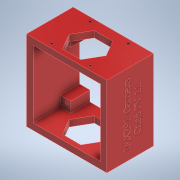
# Autodesk Inventor part: IMX291 Camera Case Base
Saved by Autodesk Inventor 2022.1 (Build 261234000, 234)
## iProperties
Created: 2021-07-23
Part Number: IMX291 Camera Case Base
Material: PET Plastic
Document SubType Name: Modeling
Designer: robst
Density: 1.541 g/cm^3
Appearance: Red
Author: robst
Autodesk Inventor part; units mm, degrees
ref_plane "YZ Plane" through (0, 0, 0) normal (1, 0, 0) x (0, 1, 0)
ref_plane "XZ Plane" through (0, 0, 0) normal (0, 1, 0) x (-1, 0, 0)
ref_plane "XY Plane" through (0, 0, 0) normal (0, 0, 1) x (1, 0, 0)
sketch "Sketch8" plane through (0, 0, 0) normal (0, 0, 1) x (1, 0, 0)
  line L0 (-17, -17) -> (17, -17) construction
  line L1 (17, -17) -> (17, 17) construction
  line L2 (17, 17) -> (-17, 17) construction
  line L3 (-17, 17) -> (-17, -17) construction
  line L4 (-17, -17) -> (17, 17) construction
  line L5 (17, -17) -> (-17, 17) construction
  circle A0 centre (-17, 17) radius 0.9
  circle A1 centre (17, 17) radius 0.9
  circle A2 centre (17, -17) radius 0.9
  circle A3 centre (-17, -17) radius 0.9
  line L6 (-21, -21) -> (21, -21)
  line L7 (21, -21) -> (21, 21)
  line L8 (21, 21) -> (-21, 21)
  line L9 (-21, 21) -> (-21, -21)
  line L10 (-21, -21) -> (21, 21) construction
  line L11 (21, -21) -> (-21, 21) construction
  line L12 (-25, -25) -> (25, -25)
  line L13 (25, -25) -> (25, 25)
  line L14 (25, 25) -> (-25, 25)
  line L15 (-25, 25) -> (-25, -25)
  line L16 (-25, -25) -> (25, 25) construction
  line L17 (25, -25) -> (-25, 25) construction
  line L18 (0, 0) -> (9.8286, 0)
  line L19 (-14.5, -14.5) -> (14.5, -14.5) construction
  line L20 (14.5, -14.5) -> (14.5, 14.5) construction
  line L21 (14.5, 14.5) -> (-14.5, 14.5) construction
  line L22 (-14.5, 14.5) -> (-14.5, -14.5) construction
  line L23 (-14.5, -14.5) -> (14.5, 14.5) construction
  line L24 (14.5, -14.5) -> (-14.5, 14.5) construction
  line L25 (-21, 21) -> (-14.5, 21)
  line L26 (-14.5, 21) -> (-14.5, 14.5)
  line L27 (-14.5, 14.5) -> (-21, 14.5)
  line L28 (-21, 14.5) -> (-21, 21)
  line L29 (21, 21) -> (14.5, 21)
  line L30 (14.5, 21) -> (14.5, 14.5)
  line L31 (14.5, 14.5) -> (21, 14.5)
  line L32 (21, 14.5) -> (21, 21)
  line L33 (21, -21) -> (14.5, -21)
  line L34 (14.5, -21) -> (14.5, -14.5)
  line L35 (14.5, -14.5) -> (21, -14.5)
  line L36 (21, -14.5) -> (21, -21)
  line L37 (-21, -21) -> (-14.5, -21)
  line L38 (-14.5, -21) -> (-14.5, -14.5)
  line L39 (-14.5, -14.5) -> (-21, -14.5)
  line L40 (-21, -14.5) -> (-21, -21)
  point P0 (-25, 0)
  point P1 (-14.5, -21)
  dimension "d46" = 34
  dimension "d47" = 34
  dimension "d48" = 1.8
  dimension "d49" = 42
  dimension "d50" = 42
  dimension "d51" = 4
  dimension "d52" = 4
  dimension "d53" = 29
  dimension "d54" = 29
  dimension "d61" = 50
  dimension "d62" = 50
  constraints: 82 end point, 16 parallel, 9 midpoint, 8 horizontal, 8 perpendicular, 4 centre point, 4 coincident, 3 equal radius, 2 point on line
  measures "d46" distance of L0.start L0.end
  measures "d47" distance of L2.end L0.start
  measures "d48" diameter of A0
  measures "d49" distance of L7.end L8.end
  measures "d50" distance of L6.end L7.end
  measures "d51" distance between parallel lines of L8 L14
  measures "d52" distance from line of point (-25, 0) L9
  measures "d53" distance of L19.start L19.end
  measures "d54" distance of L20.end L19.end
  measures "d61" distance between parallel lines of L14 L12
  measures "d62" distance between parallel lines of L15 L13
extrude "Extrusion9" add sketch "Sketch8" against normal blind 12 contours L9 L39 L38 L6 | L34 L35 L7 L6 | L9 L8 L26 L27 | L31 L30 L8 L7 | L15 L14 L13 L12
sketch "Sketch9" plane through (0, 0, 0) normal (0, 0, 1) x (1, 0, 0)
  line L0 (21, 14.5) -> (21, -14.5) projected
  line L1 (-14.5, 21) -> (14.5, 21) projected
  line L2 (-21, -14.5) -> (-21, 14.5) projected
  line L3 (14.5, -21) -> (-14.5, -21) projected
  line L4 (-25, -25) -> (25, -25) projected
  line L5 (25, -25) -> (25, 25) projected
  line L6 (25, 25) -> (-25, 25) projected
  line L7 (-25, 25) -> (-25, -25) projected
  line L8 (-21, -21) -> (21, -21)
  line L9 (21, -21) -> (21, 21)
  line L10 (21, 21) -> (-21, 21)
  line L11 (-21, 21) -> (-21, -21)
  line L12 (-21, -21) -> (21, 21) construction
  line L13 (21, -21) -> (-21, 21) construction
  line L14 (-23, -23) -> (23, -23)
  line L15 (23, -23) -> (23, 23)
  line L16 (23, 23) -> (-23, 23)
  line L17 (-23, 23) -> (-23, -23)
  line L18 (-23, -23) -> (23, 23) construction
  line L19 (23, -23) -> (-23, 23) construction
  point P0 (0, 0)
  point P1 (-14.5, -21)
  constraints: 24 end point, 4 midpoint, 4 parallel, 2 perpendicular
extrude "Extrusion10" add sketch "Sketch9" along normal blind 17 contours L7 L6 L5 L4 | L17 L16 L15 L14
sketch "Sketch10" plane through (25, -25, -12) normal (1, 0, 0) x (0, 0, -1)
  line L0 (-29, 0) -> (0, 0) construction
  line L1 (-14.5, 0) -> (-14.5, 50) construction
  line L2 (0, 50) -> (-29, 50) construction
  line L3 (-14.5, 7.4068) -> (-14.5, 5.8574)
  line L4 (-14.5, 5.8574) -> (-14.9084, 5.8574)
  line L5 (-14.9084, 5.8574) -> (-14.9084, 6.3663)
  line L6 (-14.9084, 6.3663) -> (-18.0916, 6.3663)
  line L7 (-18.0916, 6.3663) -> (-18.0916, 5.8574)
  line L8 (-18.0916, 5.8574) -> (-18.5, 5.8574)
  line L9 (-18.5, 5.8574) -> (-18.5, 7.4068)
  line L10 (-18.5, 7.4068) -> (-18.0916, 7.4068)
  line L11 (-18.0916, 7.4068) -> (-18.0916, 6.8979)
  line L12 (-18.0916, 6.8979) -> (-14.9084, 6.8979)
  line L13 (-14.9084, 6.8979) -> (-14.9084, 7.4068)
  line L14 (-14.9084, 7.4068) -> (-14.5, 7.4068)
  line L15 (-14.5, 11.4943) -> (-14.5, 10.9627)
  line L16 (-14.5, 10.9627) -> (-17.9457, 10.9627)
  line L17 (-17.9457, 10.9627) -> (-15.6021, 9.919)
  line L18 (-15.6021, 9.919) -> (-15.6021, 9.5948)
  line L19 (-15.6021, 9.5948) -> (-17.9457, 8.5608)
  line L20 (-17.9457, 8.5608) -> (-14.5, 8.5608)
  line L21 (-14.5, 8.5608) -> (-14.5, 8.0648)
  line L22 (-14.5, 8.0648) -> (-18.5, 8.0648)
  line L23 (-18.5, 8.0648) -> (-18.5, 8.7909)
  line L24 (-18.5, 8.7909) -> (-16.2731, 9.7893)
  line L25 (-16.2731, 9.7893) -> (-18.5, 10.7553)
  line L26 (-18.5, 10.7553) -> (-18.5, 11.4943)
  line L27 (-18.5, 11.4943) -> (-14.5, 11.4943)
  line L28 (-14.5, 15.0697) -> (-14.5, 14.4603)
  line L29 (-14.5, 14.4603) -> (-16.0948, 13.4878)
  line L30 (-16.0948, 13.4878) -> (-14.5, 12.4959)
  line L31 (-14.5, 12.4959) -> (-14.5, 11.9222)
  line L32 (-14.5, 11.9222) -> (-16.5032, 13.1961)
  line L33 (-16.5032, 13.1961) -> (-18.5, 11.9611)
  line L34 (-18.5, 11.9611) -> (-18.5, 12.5705)
  line L35 (-18.5, 12.5705) -> (-16.9344, 13.5235)
  line L36 (-16.9344, 13.5235) -> (-18.5, 14.4959)
  line L37 (-18.5, 14.4959) -> (-18.5, 15.0697)
  line L38 (-18.5, 15.0697) -> (-16.5292, 13.8185)
  line L39 (-16.5292, 13.8185) -> (-14.5, 15.0697)
  line L40 (-14.5, 17.8509) -> (-14.5, 15.3841)
  line L41 (-14.5, 15.3841) -> (-15.0673, 15.3841)
  spline S0 degree 2 poles (-15.0673, 15.3841) (-15.3169, 15.6499) (-15.7804, 16.1232) (-16.03, 16.3501) knots 0 0 0 1 2 2 2
  spline S1 degree 2 poles (-16.03, 16.3501) (-16.5324, 16.8071) (-17.1353, 17.141) (-17.4562, 17.141) knots 0 0 0 1 2 2 2
  spline S2 degree 2 poles (-17.4562, 17.141) (-17.6248, 17.141) (-17.8776, 17.0373) (-17.9587, 16.9433) knots 0 0 0 1 2 2 2
  spline S3 degree 2 poles (-17.9587, 16.9433) (-18.0397, 16.8493) (-18.1207, 16.6029) (-18.1207, 16.4538) knots 0 0 0 1 2 2 2
  spline S4 degree 2 poles (-18.1207, 16.4538) (-18.1207, 16.3112) (-18.0494, 16.0194) (-17.9943, 15.8865) knots 0 0 0 1 2 2 2
  spline S5 degree 2 poles (-17.9943, 15.8865) (-17.9489, 15.7731) (-17.8193, 15.5624) (-17.7739, 15.4976) knots 0 0 0 1 2 2 2
  line L42 (-17.7739, 15.4976) -> (-17.7739, 15.4684)
  line L43 (-17.7739, 15.4684) -> (-18.3444, 15.4684)
  spline S6 degree 2 poles (-18.3444, 15.4684) (-18.4254, 15.6337) (-18.5843, 16.2269) (-18.5843, 16.4927) knots 0 0 0 1 2 2 2
  spline S7 degree 2 poles (-18.5843, 16.4927) (-18.5843, 17.0535) (-17.9911, 17.6856) (-17.4854, 17.6856) knots 0 0 0 1 2 2 2
  spline S8 degree 2 poles (-17.4854, 17.6856) (-17.2488, 17.6856) (-16.8533, 17.5754) (-16.6848, 17.4781) knots 0 0 0 1 2 2 2
  spline S9 degree 2 poles (-16.6848, 17.4781) (-16.5097, 17.3809) (-16.1661, 17.0989) (-16.0008, 16.9433) knots 0 0 0 1 2 2 2
  spline S10 degree 2 poles (-16.0008, 16.9433) (-15.7253, 16.6904) (-15.1353, 16.0713) (-14.9635, 15.8865) knots 0 0 0 1 2 2 2
  line L44 (-14.9635, 15.8865) -> (-14.9635, 17.8509)
  line L45 (-14.9635, 17.8509) -> (-14.5, 17.8509)
  spline S11 degree 2 poles (-17.2002, 18.2755) (-17.5081, 18.2755) (-18.0203, 18.4765) (-18.205, 18.6515) knots 0 0 0 1 2 2 2
  spline S12 degree 2 poles (-18.205, 18.6515) (-18.3833, 18.8169) (-18.581, 19.2998) (-18.581, 19.5462) knots 0 0 0 1 2 2 2
  spline S13 degree 2 poles (-18.581, 19.5462) (-18.581, 19.8217) (-18.3963, 20.269) (-18.2212, 20.4344) knots 0 0 0 1 2 2 2
  spline S14 degree 2 poles (-18.2212, 20.4344) (-18.0008, 20.6418) (-17.2877, 20.8687) (-16.7399, 20.8687) knots 0 0 0 1 2 2 2
  spline S15 degree 2 poles (-16.7399, 20.8687) (-16.2439, 20.8687) (-15.3558, 20.6451) (-15.0608, 20.4279) knots 0 0 0 1 2 2 2
  spline S16 degree 2 poles (-15.0608, 20.4279) (-14.7496, 20.1977) (-14.4222, 19.5494) (-14.4222, 19.0762) knots 0 0 0 1 2 2 2
  spline S17 degree 2 poles (-14.4222, 19.0762) (-14.4222, 18.9692) (-14.4449, 18.7261) (-14.4773, 18.6224) knots 0 0 0 1 2 2 2
  line L46 (-14.4773, 18.6224) -> (-14.9927, 18.6224)
  line L47 (-14.9927, 18.6224) -> (-14.9927, 18.6483)
  spline S18 degree 2 poles (-14.9927, 18.6483) (-14.9538, 18.7164) (-14.8857, 19.0016) (-14.8857, 19.1475) knots 0 0 0 1 2 2 2
  spline S19 degree 2 poles (-14.8857, 19.1475) (-14.8857, 19.6726) (-15.5794, 20.2723) (-16.2212, 20.3144) knots 0 0 0 1 2 2 2
  spline S20 degree 2 poles (-16.2212, 20.3144) (-16.0754, 20.1005) (-15.9425, 19.7115) (-15.9425, 19.4814) knots 0 0 0 1 2 2 2
  spline S21 degree 2 poles (-15.9425, 19.4814) (-15.9425, 19.2609) (-16.0397, 18.8947) (-16.1791, 18.7099) knots 0 0 0 1 2 2 2
  spline S22 degree 2 poles (-16.1791, 18.7099) (-16.3444, 18.4959) (-16.8468, 18.2755) (-17.2002, 18.2755) knots 0 0 0 1 2 2 2
  spline S23 degree 2 poles (-16.8598, 20.3274) (-17.265, 20.3274) (-17.7771, 20.1783) (-17.9165, 20.0454) knots 0 0 0 1 2 2 2
  spline S24 degree 2 poles (-17.9165, 20.0454) (-18.0462, 19.9287) (-18.1434, 19.6856) (-18.1434, 19.5429) knots 0 0 0 1 2 2 2
  spline S25 degree 2 poles (-18.1434, 19.5429) (-18.1434, 19.2123) (-17.6702, 18.8201) (-17.2229, 18.8201) knots 0 0 0 1 2 2 2
  spline S26 degree 2 poles (-17.2229, 18.8201) (-16.97, 18.8201) (-16.6426, 18.9498) (-16.5259, 19.0924) knots 0 0 0 1 2 2 2
  spline S27 degree 2 poles (-16.5259, 19.0924) (-16.4417, 19.1961) (-16.3865, 19.4522) (-16.3865, 19.6013) knots 0 0 0 1 2 2 2
  spline S28 degree 2 poles (-16.3865, 19.6013) (-16.3865, 19.7731) (-16.5065, 20.1686) (-16.607, 20.3177) knots 0 0 0 1 2 2 2
  spline S29 degree 2 poles (-16.607, 20.3177) (-16.6459, 20.3209) (-16.7788, 20.3274) (-16.8598, 20.3274) knots 0 0 0 1 2 2 2
  line L48 (-14.5, 23.6532) -> (-14.5, 21.7018)
  line L49 (-14.5, 21.7018) -> (-14.9084, 21.7018)
  line L50 (-14.9084, 21.7018) -> (-14.9084, 22.4279)
  line L51 (-14.9084, 22.4279) -> (-17.5891, 22.4279)
  line L52 (-17.5891, 22.4279) -> (-17.5891, 21.7018)
  line L53 (-17.5891, 21.7018) -> (-17.9554, 21.7018)
  spline S30 degree 2 poles (-17.9554, 21.7018) (-17.9554, 22.1135) (-18.1888, 22.5024) (-18.513, 22.5284) knots 0 0 0 1 2 2 2
  line L54 (-18.513, 22.5284) -> (-18.513, 22.9433)
  line L55 (-18.513, 22.9433) -> (-14.9084, 22.9433)
  line L56 (-14.9084, 22.9433) -> (-14.9084, 23.6532)
  line L57 (-14.9084, 23.6532) -> (-14.5, 23.6532)
  spline S31 degree 2 poles (-14.4287, 27.7828) (-14.4287, 27.3938) (-14.6912, 26.7358) (-14.9538, 26.4959) knots 0 0 0 1 2 2 2
  spline S32 degree 2 poles (-14.9538, 26.4959) (-15.2131, 26.2561) (-15.9911, 25.9935) (-16.4968, 25.9935) knots 0 0 0 1 2 2 2
  spline S33 degree 2 poles (-16.4968, 25.9935) (-16.9992, 25.9935) (-17.7447, 26.2496) (-18.0203, 26.4927) knots 0 0 0 1 2 2 2
  spline S34 degree 2 poles (-18.0203, 26.4927) (-18.2893, 26.7326) (-18.5713, 27.3874) (-18.5713, 27.7925) knots 0 0 0 1 2 2 2
  spline S35 degree 2 poles (-18.5713, 27.7925) (-18.5713, 27.9935) (-18.513, 28.3468) (-18.4676, 28.4959) knots 0 0 0 1 2 2 2
  spline S36 degree 2 poles (-18.4676, 28.4959) (-18.4254, 28.6256) (-18.3055, 28.8947) (-18.2342, 29.0276) knots 0 0 0 1 2 2 2
  line L58 (-18.2342, 29.0276) -> (-17.5924, 29.0276)
  line L59 (-17.5924, 29.0276) -> (-17.5924, 28.9854)
  spline S37 degree 2 poles (-17.5924, 28.9854) (-17.6572, 28.9141) (-17.8387, 28.6937) (-17.9263, 28.5348) knots 0 0 0 1 2 2 2
  spline S38 degree 2 poles (-17.9263, 28.5348) (-18.0105, 28.3825) (-18.1175, 28.0227) (-18.1175, 27.7893) knots 0 0 0 1 2 2 2
  spline S39 degree 2 poles (-18.1175, 27.7893) (-18.1175, 27.5332) (-17.9068, 27.0762) (-17.7058, 26.9044) knots 0 0 0 1 2 2 2
  spline S40 degree 2 poles (-17.7058, 26.9044) (-17.5016, 26.7358) (-16.8825, 26.5478) (-16.4968, 26.5478) knots 0 0 0 1 2 2 2
  spline S41 degree 2 poles (-16.4968, 26.5478) (-16.0851, 26.5478) (-15.4919, 26.7455) (-15.2877, 26.9173) knots 0 0 0 1 2 2 2
  spline S42 degree 2 poles (-15.2877, 26.9173) (-15.09, 27.0859) (-14.889, 27.5365) (-14.889, 27.7893) knots 0 0 0 1 2 2 2
  spline S43 degree 2 poles (-14.889, 27.7893) (-14.889, 28.0194) (-15.0024, 28.4117) (-15.0867, 28.564) knots 0 0 0 1 2 2 2
  spline S44 degree 2 poles (-15.0867, 28.564) (-15.171, 28.7099) (-15.346, 28.9271) (-15.4076, 28.9887) knots 0 0 0 1 2 2 2
  line L60 (-15.4076, 28.9887) -> (-15.4076, 29.0276)
  line L61 (-15.4076, 29.0276) -> (-14.7723, 29.0276)
  spline S45 degree 2 poles (-14.7723, 29.0276) (-14.7107, 28.8947) (-14.5972, 28.6613) (-14.5454, 28.4959) knots 0 0 0 1 2 2 2
  spline S46 degree 2 poles (-14.5454, 28.4959) (-14.487, 28.3209) (-14.4287, 28.0227) (-14.4287, 27.7828) knots 0 0 0 1 2 2 2
  spline S47 degree 2 poles (-14.8177, 31.1572) (-14.7723, 31.0956) (-14.6102, 30.8882) (-14.5616, 30.7909) knots 0 0 0 1 2 2 2
  spline S48 degree 2 poles (-14.5616, 30.7909) (-14.4903, 30.658) (-14.4157, 30.4084) (-14.4157, 30.1815) knots 0 0 0 1 2 2 2
  spline S49 degree 2 poles (-14.4157, 30.1815) (-14.4157, 29.9968) (-14.5551, 29.6629) (-14.6815, 29.5365) knots 0 0 0 1 2 2 2
  spline S50 degree 2 poles (-14.6815, 29.5365) (-14.8047, 29.4165) (-15.1677, 29.2707) (-15.3687, 29.2707) knots 0 0 0 1 2 2 2
  spline S51 degree 2 poles (-15.3687, 29.2707) (-15.6799, 29.2707) (-16.1207, 29.5332) (-16.2472, 29.8185) knots 0 0 0 1 2 2 2
  spline S52 degree 2 poles (-16.2472, 29.8185) (-16.3639, 30.0713) (-16.4514, 30.7585) (-16.4741, 31.1572) knots 0 0 0 1 2 2 2
  line L62 (-16.4741, 31.1572) -> (-16.5713, 31.1572)
  spline S53 degree 2 poles (-16.5713, 31.1572) (-16.7464, 31.1572) (-16.9635, 31.0502) (-17.0251, 30.953) knots 0 0 0 1 2 2 2
  spline S54 degree 2 poles (-17.0251, 30.953) (-17.0867, 30.8558) (-17.1256, 30.577) (-17.1256, 30.4279) knots 0 0 0 1 2 2 2
  spline S55 degree 2 poles (-17.1256, 30.4279) (-17.1256, 30.2528) (-17.0219, 29.7796) (-16.9214, 29.543) knots 0 0 0 1 2 2 2
  line L63 (-16.9214, 29.543) -> (-16.9214, 29.5138)
  line L64 (-16.9214, 29.5138) -> (-17.4368, 29.5138)
  spline S56 degree 2 poles (-17.4368, 29.5138) (-17.4757, 29.6532) (-17.5729, 30.175) (-17.5729, 30.4311) knots 0 0 0 1 2 2 2
  spline S57 degree 2 poles (-17.5729, 30.4311) (-17.5729, 30.7423) (-17.4757, 31.1669) (-17.3493, 31.3355) knots 0 0 0 1 2 2 2
  spline S58 degree 2 poles (-17.3493, 31.3355) (-17.2261, 31.5008) (-16.8339, 31.6629) (-16.5519, 31.6629) knots 0 0 0 1 2 2 2
  line L65 (-16.5519, 31.6629) -> (-14.5, 31.6629)
  line L66 (-14.5, 31.6629) -> (-14.5, 31.1572)
  line L67 (-14.5, 31.1572) -> (-14.8177, 31.1572)
  line L68 (-15.2391, 31.1572) -> (-16.0721, 31.1572)
  spline S59 degree 2 poles (-16.0721, 31.1572) (-16.0559, 30.9757) (-16.0008, 30.4279) (-15.9489, 30.2561) knots 0 0 0 1 2 2 2
  spline S60 degree 2 poles (-15.9489, 30.2561) (-15.8874, 30.0551) (-15.6313, 29.7925) (-15.4044, 29.7925) knots 0 0 0 1 2 2 2
  spline S61 degree 2 poles (-15.4044, 29.7925) (-15.1451, 29.7925) (-14.8825, 30.0843) (-14.8825, 30.363) knots 0 0 0 1 2 2 2
  spline S62 degree 2 poles (-14.8825, 30.363) (-14.8825, 30.5997) (-15.0867, 30.9887) (-15.2391, 31.1572) knots 0 0 0 1 2 2 2
  line L69 (-14.5, 35.7763) -> (-16.2374, 35.7763)
  spline S63 degree 2 poles (-16.2374, 35.7763) (-16.4449, 35.7763) (-16.7982, 35.7439) (-16.8955, 35.6921) knots 0 0 0 1 2 2 2
  spline S64 degree 2 poles (-16.8955, 35.6921) (-17.0024, 35.6402) (-17.1062, 35.4425) (-17.1062, 35.2707) knots 0 0 0 1 2 2 2
  spline S65 degree 2 poles (-17.1062, 35.2707) (-17.1062, 35.1151) (-16.9149, 34.7585) (-16.7334, 34.5705) knots 0 0 0 1 2 2 2
  spline S66 degree 2 poles (-16.7334, 34.5705) (-16.688, 34.5737) (-16.5616, 34.5802) (-16.4773, 34.5802) knots 0 0 0 1 2 2 2
  line L70 (-16.4773, 34.5802) -> (-14.5, 34.5802)
  line L71 (-14.5, 34.5802) -> (-14.5, 34.0746)
  line L72 (-14.5, 34.0746) -> (-16.2374, 34.0746)
  spline S67 degree 2 poles (-16.2374, 34.0746) (-16.4449, 34.0746) (-16.7982, 34.0421) (-16.8955, 33.9903) knots 0 0 0 1 2 2 2
  spline S68 degree 2 poles (-16.8955, 33.9903) (-17.0024, 33.9384) (-17.1062, 33.7407) (-17.1062, 33.5689) knots 0 0 0 1 2 2 2
  spline S69 degree 2 poles (-17.1062, 33.5689) (-17.1062, 33.4068) (-16.9019, 33.047) (-16.7431, 32.8784) knots 0 0 0 1 2 2 2
  line L73 (-16.7431, 32.8784) -> (-14.5, 32.8784)
  line L74 (-14.5, 32.8784) -> (-14.5, 32.3728)
  line L75 (-14.5, 32.3728) -> (-17.5016, 32.3728)
  line L76 (-17.5016, 32.3728) -> (-17.5016, 32.8784)
  line L77 (-17.5016, 32.8784) -> (-17.171, 32.8784)
  spline S70 degree 2 poles (-17.171, 32.8784) (-17.3687, 33.0762) (-17.5859, 33.4652) (-17.5859, 33.6985) knots 0 0 0 1 2 2 2
  spline S71 degree 2 poles (-17.5859, 33.6985) (-17.5859, 33.9643) (-17.3428, 34.376) (-17.0673, 34.483) knots 0 0 0 1 2 2 2
  spline S72 degree 2 poles (-17.0673, 34.483) (-17.3233, 34.7131) (-17.5859, 35.1475) (-17.5859, 35.4003) knots 0 0 0 1 2 2 2
  spline S73 degree 2 poles (-17.5859, 35.4003) (-17.5859, 35.5948) (-17.466, 35.9125) (-17.3298, 36.0292) knots 0 0 0 1 2 2 2
  spline S74 degree 2 poles (-17.3298, 36.0292) (-17.1937, 36.1491) (-16.7853, 36.282) (-16.4773, 36.282) knots 0 0 0 1 2 2 2
  line L78 (-16.4773, 36.282) -> (-14.5, 36.282)
  line L79 (-14.5, 36.282) -> (-14.5, 35.7763)
  spline S75 degree 2 poles (-14.4319, 38.295) (-14.4319, 37.5754) (-15.2391, 36.7844) (-15.9846, 36.7844) knots 0 0 0 1 2 2 2
  spline S76 degree 2 poles (-15.9846, 36.7844) (-16.7172, 36.7844) (-17.5859, 37.5527) (-17.5859, 38.1718) knots 0 0 0 1 2 2 2
  spline S77 degree 2 poles (-17.5859, 38.1718) (-17.5859, 38.4506) (-17.4238, 38.8817) (-17.252, 39.0405) knots 0 0 0 1 2 2 2
  spline S78 degree 2 poles (-17.252, 39.0405) (-17.0802, 39.2026) (-16.5843, 39.3744) (-16.2245, 39.3744) knots 0 0 0 1 2 2 2
  line L80 (-16.2245, 39.3744) -> (-15.9489, 39.3744)
  line L81 (-15.9489, 39.3744) -> (-15.9489, 37.2966)
  spline S79 degree 2 poles (-15.9489, 37.2966) (-15.4271, 37.2966) (-14.8728, 37.8217) (-14.8728, 38.2885) knots 0 0 0 1 2 2 2
  spline S80 degree 2 poles (-14.8728, 38.2885) (-14.8728, 38.4538) (-14.9473, 38.7747) (-15.0057, 38.9044) knots 0 0 0 1 2 2 2
  spline S81 degree 2 poles (-15.0057, 38.9044) (-15.0705, 39.0405) (-15.184, 39.2285) (-15.2358, 39.2901) knots 0 0 0 1 2 2 2
  line L82 (-15.2358, 39.2901) -> (-15.2358, 39.3193)
  line L83 (-15.2358, 39.3193) -> (-14.6848, 39.3193)
  spline S82 degree 2 poles (-14.6848, 39.3193) (-14.6491, 39.2318) (-14.5454, 38.966) (-14.5162, 38.8622) knots 0 0 0 1 2 2 2
  spline S83 degree 2 poles (-14.5162, 38.8622) (-14.4741, 38.7164) (-14.4319, 38.4765) (-14.4319, 38.295) knots 0 0 0 1 2 2 2
  spline S84 degree 2 poles (-16.3347, 38.8817) (-16.5389, 38.8752) (-16.8371, 38.7909) (-16.9376, 38.7099) knots 0 0 0 1 2 2 2
  spline S85 degree 2 poles (-16.9376, 38.7099) (-17.0511, 38.6224) (-17.171, 38.3468) (-17.171, 38.1426) knots 0 0 0 1 2 2 2
  spline S86 degree 2 poles (-17.171, 38.1426) (-17.171, 37.9417) (-17.0511, 37.6596) (-16.9344, 37.543) knots 0 0 0 1 2 2 2
  spline S87 degree 2 poles (-16.9344, 37.543) (-16.8144, 37.4295) (-16.5259, 37.3128) (-16.3347, 37.2966) knots 0 0 0 1 2 2 2
  line L84 (-16.3347, 37.2966) -> (-16.3347, 38.8817)
  line L85 (-16.9603, 41.4781) -> (-16.9603, 41.4522)
  spline S88 degree 2 poles (-16.9603, 41.4522) (-16.9765, 41.3938) (-16.983, 41.2674) (-16.983, 41.1799) knots 0 0 0 1 2 2 2
  spline S89 degree 2 poles (-16.983, 41.1799) (-16.983, 40.9757) (-16.8047, 40.5737) (-16.6297, 40.3922) knots 0 0 0 1 2 2 2
  line L86 (-16.6297, 40.3922) -> (-14.5, 40.3922)
  line L87 (-14.5, 40.3922) -> (-14.5, 39.8865)
  line L88 (-14.5, 39.8865) -> (-17.5016, 39.8865)
  line L89 (-17.5016, 39.8865) -> (-17.5016, 40.3922)
  line L90 (-17.5016, 40.3922) -> (-17.0543, 40.3922)
  spline S90 degree 2 poles (-17.0543, 40.3922) (-17.3006, 40.6677) (-17.5016, 41.0794) (-17.5016, 41.2739) knots 0 0 0 1 2 2 2
  spline S91 degree 2 poles (-17.5016, 41.2739) (-17.5016, 41.3517) (-17.4951, 41.4295) (-17.4854, 41.4781) knots 0 0 0 1 2 2 2
  line L91 (-17.4854, 41.4781) -> (-16.9603, 41.4781)
  spline S92 degree 2 poles (-14.8177, 43.543) (-14.7723, 43.4814) (-14.6102, 43.2739) (-14.5616, 43.1767) knots 0 0 0 1 2 2 2
  spline S93 degree 2 poles (-14.5616, 43.1767) (-14.4903, 43.0438) (-14.4157, 42.7942) (-14.4157, 42.5673) knots 0 0 0 1 2 2 2
  spline S94 degree 2 poles (-14.4157, 42.5673) (-14.4157, 42.3825) (-14.5551, 42.0486) (-14.6815, 41.9222) knots 0 0 0 1 2 2 2
  spline S95 degree 2 poles (-14.6815, 41.9222) (-14.8047, 41.8023) (-15.1677, 41.6564) (-15.3687, 41.6564) knots 0 0 0 1 2 2 2
  spline S96 degree 2 poles (-15.3687, 41.6564) (-15.6799, 41.6564) (-16.1207, 41.919) (-16.2472, 42.2042) knots 0 0 0 1 2 2 2
  spline S97 degree 2 poles (-16.2472, 42.2042) (-16.3639, 42.4571) (-16.4514, 43.1442) (-16.4741, 43.543) knots 0 0 0 1 2 2 2
  line L92 (-16.4741, 43.543) -> (-16.5713, 43.543)
  spline S98 degree 2 poles (-16.5713, 43.543) (-16.7464, 43.543) (-16.9635, 43.436) (-17.0251, 43.3387) knots 0 0 0 1 2 2 2
  spline S99 degree 2 poles (-17.0251, 43.3387) (-17.0867, 43.2415) (-17.1256, 42.9627) (-17.1256, 42.8136) knots 0 0 0 1 2 2 2
  spline S100 degree 2 poles (-17.1256, 42.8136) (-17.1256, 42.6386) (-17.0219, 42.1653) (-16.9214, 41.9287) knots 0 0 0 1 2 2 2
  line L93 (-16.9214, 41.9287) -> (-16.9214, 41.8995)
  line L94 (-16.9214, 41.8995) -> (-17.4368, 41.8995)
  spline S101 degree 2 poles (-17.4368, 41.8995) (-17.4757, 42.0389) (-17.5729, 42.5608) (-17.5729, 42.8169) knots 0 0 0 1 2 2 2
  spline S102 degree 2 poles (-17.5729, 42.8169) (-17.5729, 43.128) (-17.4757, 43.5527) (-17.3493, 43.7212) knots 0 0 0 1 2 2 2
  spline S103 degree 2 poles (-17.3493, 43.7212) (-17.2261, 43.8865) (-16.8339, 44.0486) (-16.5519, 44.0486) knots 0 0 0 1 2 2 2
  line L95 (-16.5519, 44.0486) -> (-14.5, 44.0486)
  line L96 (-14.5, 44.0486) -> (-14.5, 43.543)
  line L97 (-14.5, 43.543) -> (-14.8177, 43.543)
  line L98 (-15.2391, 43.543) -> (-16.0721, 43.543)
  spline S104 degree 2 poles (-16.0721, 43.543) (-16.0559, 43.3614) (-16.0008, 42.8136) (-15.9489, 42.6418) knots 0 0 0 1 2 2 2
  spline S105 degree 2 poles (-15.9489, 42.6418) (-15.8874, 42.4408) (-15.6313, 42.1783) (-15.4044, 42.1783) knots 0 0 0 1 2 2 2
  spline S106 degree 2 poles (-15.4044, 42.1783) (-15.1451, 42.1783) (-14.8825, 42.47) (-14.8825, 42.7488) knots 0 0 0 1 2 2 2
  spline S107 degree 2 poles (-14.8825, 42.7488) (-14.8825, 42.9854) (-15.0867, 43.3744) (-15.2391, 43.543) knots 0 0 0 1 2 2 2
  spline S108 degree 2 poles (-7.8362, 13.3193) (-7.8362, 12.9303) (-8.0988, 12.2723) (-8.3613, 12.0324) knots 0 0 0 1 2 2 2
  spline S109 degree 2 poles (-8.3613, 12.0324) (-8.6207, 11.7925) (-9.3986, 11.53) (-9.9043, 11.53) knots 0 0 0 1 2 2 2
  spline S110 degree 2 poles (-9.9043, 11.53) (-10.4067, 11.53) (-11.1523, 11.7861) (-11.4278, 12.0292) knots 0 0 0 1 2 2 2
  spline S111 degree 2 poles (-11.4278, 12.0292) (-11.6968, 12.269) (-11.9788, 12.9238) (-11.9788, 13.329) knots 0 0 0 1 2 2 2
  spline S112 degree 2 poles (-11.9788, 13.329) (-11.9788, 13.53) (-11.9205, 13.8833) (-11.8751, 14.0324) knots 0 0 0 1 2 2 2
  spline S113 degree 2 poles (-11.8751, 14.0324) (-11.833, 14.1621) (-11.713, 14.4311) (-11.6417, 14.564) knots 0 0 0 1 2 2 2
  line L99 (-11.6417, 14.564) -> (-10.9999, 14.564)
  line L100 (-10.9999, 14.564) -> (-10.9999, 14.5219)
  spline S114 degree 2 poles (-10.9999, 14.5219) (-11.0647, 14.4506) (-11.2463, 14.2301) (-11.3338, 14.0713) knots 0 0 0 1 2 2 2
  spline S115 degree 2 poles (-11.3338, 14.0713) (-11.4181, 13.919) (-11.525, 13.5592) (-11.525, 13.3258) knots 0 0 0 1 2 2 2
  spline S116 degree 2 poles (-11.525, 13.3258) (-11.525, 13.0697) (-11.3143, 12.6126) (-11.1134, 12.4408) knots 0 0 0 1 2 2 2
  spline S117 degree 2 poles (-11.1134, 12.4408) (-10.9091, 12.2723) (-10.29, 12.0843) (-9.9043, 12.0843) knots 0 0 0 1 2 2 2
  spline S118 degree 2 poles (-9.9043, 12.0843) (-9.4926, 12.0843) (-8.8994, 12.282) (-8.6952, 12.4538) knots 0 0 0 1 2 2 2
  spline S119 degree 2 poles (-8.6952, 12.4538) (-8.4975, 12.6224) (-8.2965, 13.0729) (-8.2965, 13.3258) knots 0 0 0 1 2 2 2
  spline S120 degree 2 poles (-8.2965, 13.3258) (-8.2965, 13.5559) (-8.41, 13.9481) (-8.4942, 14.1005) knots 0 0 0 1 2 2 2
  spline S121 degree 2 poles (-8.4942, 14.1005) (-8.5785, 14.2464) (-8.7536, 14.4635) (-8.8151, 14.5251) knots 0 0 0 1 2 2 2
  line L101 (-8.8151, 14.5251) -> (-8.8151, 14.564)
  line L102 (-8.8151, 14.564) -> (-8.1798, 14.564)
  spline S122 degree 2 poles (-8.1798, 14.564) (-8.1182, 14.4311) (-8.0048, 14.1977) (-7.9529, 14.0324) knots 0 0 0 1 2 2 2
  spline S123 degree 2 poles (-7.9529, 14.0324) (-7.8946, 13.8574) (-7.8362, 13.5592) (-7.8362, 13.3193) knots 0 0 0 1 2 2 2
  spline S124 degree 2 poles (-8.2252, 16.6937) (-8.1798, 16.6321) (-8.0177, 16.4246) (-7.9691, 16.3274) knots 0 0 0 1 2 2 2
  spline S125 degree 2 poles (-7.9691, 16.3274) (-7.8978, 16.1945) (-7.8233, 15.9449) (-7.8233, 15.718) knots 0 0 0 1 2 2 2
  spline S126 degree 2 poles (-7.8233, 15.718) (-7.8233, 15.5332) (-7.9626, 15.1994) (-8.0891, 15.0729) knots 0 0 0 1 2 2 2
  spline S127 degree 2 poles (-8.0891, 15.0729) (-8.2122, 14.953) (-8.5753, 14.8071) (-8.7762, 14.8071) knots 0 0 0 1 2 2 2
  spline S128 degree 2 poles (-8.7762, 14.8071) (-9.0874, 14.8071) (-9.5283, 15.0697) (-9.6547, 15.3549) knots 0 0 0 1 2 2 2
  spline S129 degree 2 poles (-9.6547, 15.3549) (-9.7714, 15.6078) (-9.8589, 16.295) (-9.8816, 16.6937) knots 0 0 0 1 2 2 2
  line L103 (-9.8816, 16.6937) -> (-9.9788, 16.6937)
  spline S130 degree 2 poles (-9.9788, 16.6937) (-10.1539, 16.6937) (-10.3711, 16.5867) (-10.4327, 16.4895) knots 0 0 0 1 2 2 2
  spline S131 degree 2 poles (-10.4327, 16.4895) (-10.4942, 16.3922) (-10.5331, 16.1135) (-10.5331, 15.9643) knots 0 0 0 1 2 2 2
  spline S132 degree 2 poles (-10.5331, 15.9643) (-10.5331, 15.7893) (-10.4294, 15.316) (-10.3289, 15.0794) knots 0 0 0 1 2 2 2
  line L104 (-10.3289, 15.0794) -> (-10.3289, 15.0502)
  line L105 (-10.3289, 15.0502) -> (-10.8443, 15.0502)
  spline S133 degree 2 poles (-10.8443, 15.0502) (-10.8832, 15.1896) (-10.9805, 15.7115) (-10.9805, 15.9676) knots 0 0 0 1 2 2 2
  spline S134 degree 2 poles (-10.9805, 15.9676) (-10.9805, 16.2788) (-10.8832, 16.7034) (-10.7568, 16.872) knots 0 0 0 1 2 2 2
  spline S135 degree 2 poles (-10.7568, 16.872) (-10.6336, 17.0373) (-10.2414, 17.1994) (-9.9594, 17.1994) knots 0 0 0 1 2 2 2
  line L106 (-9.9594, 17.1994) -> (-7.9075, 17.1994)
  line L107 (-7.9075, 17.1994) -> (-7.9075, 16.6937)
  line L108 (-7.9075, 16.6937) -> (-8.2252, 16.6937)
  line L109 (-8.6466, 16.6937) -> (-9.4797, 16.6937)
  spline S136 degree 2 poles (-9.4797, 16.6937) (-9.4634, 16.5122) (-9.4083, 15.9643) (-9.3565, 15.7925) knots 0 0 0 1 2 2 2
  spline S137 degree 2 poles (-9.3565, 15.7925) (-9.2949, 15.5916) (-9.0388, 15.329) (-8.8119, 15.329) knots 0 0 0 1 2 2 2
  spline S138 degree 2 poles (-8.8119, 15.329) (-8.5526, 15.329) (-8.29, 15.6207) (-8.29, 15.8995) knots 0 0 0 1 2 2 2
  spline S139 degree 2 poles (-8.29, 15.8995) (-8.29, 16.1361) (-8.4942, 16.5251) (-8.6466, 16.6937) knots 0 0 0 1 2 2 2
  spline S140 degree 2 poles (-7.8362, 18.7196) (-7.8362, 18.4182) (-7.9983, 17.8963) (-8.0891, 17.7245) knots 0 0 0 1 2 2 2
  line L110 (-8.0891, 17.7245) -> (-8.6563, 17.7245)
  line L111 (-8.6563, 17.7245) -> (-8.6563, 17.7504)
  spline S141 degree 2 poles (-8.6563, 17.7504) (-8.6044, 17.8152) (-8.4813, 17.9903) (-8.4132, 18.1361) knots 0 0 0 1 2 2 2
  spline S142 degree 2 poles (-8.4132, 18.1361) (-8.3516, 18.2626) (-8.2609, 18.5737) (-8.2609, 18.7391) knots 0 0 0 1 2 2 2
  spline S143 degree 2 poles (-8.2609, 18.7391) (-8.2609, 18.859) (-8.316, 19.1345) (-8.3613, 19.1994) knots 0 0 0 1 2 2 2
  spline S144 degree 2 poles (-8.3613, 19.1994) (-8.4229, 19.2934) (-8.5623, 19.3776) (-8.7049, 19.3776) knots 0 0 0 1 2 2 2
  spline S145 degree 2 poles (-8.7049, 19.3776) (-8.8832, 19.3776) (-9.068, 19.1831) (-9.1296, 18.9335) knots 0 0 0 1 2 2 2
  spline S146 degree 2 poles (-9.1296, 18.9335) (-9.1523, 18.8363) (-9.2171, 18.5251) (-9.2527, 18.3922) knots 0 0 0 1 2 2 2
  spline S147 degree 2 poles (-9.2527, 18.3922) (-9.3532, 18.0486) (-9.7681, 17.7374) (-10.0631, 17.7374) knots 0 0 0 1 2 2 2
  spline S148 degree 2 poles (-10.0631, 17.7374) (-10.4715, 17.7374) (-10.9805, 18.3501) (-10.9805, 18.8558) knots 0 0 0 1 2 2 2
  spline S149 degree 2 poles (-10.9805, 18.8558) (-10.9805, 19.1053) (-10.8573, 19.611) (-10.7633, 19.7828) knots 0 0 0 1 2 2 2
  line L112 (-10.7633, 19.7828) -> (-10.222, 19.7828)
  line L113 (-10.222, 19.7828) -> (-10.222, 19.7569)
  spline S150 degree 2 poles (-10.222, 19.7569) (-10.3775, 19.5624) (-10.5558, 19.0891) (-10.5558, 18.846) knots 0 0 0 1 2 2 2
  spline S151 degree 2 poles (-10.5558, 18.846) (-10.5558, 18.5964) (-10.3451, 18.2528) (-10.1344, 18.2528) knots 0 0 0 1 2 2 2
  spline S152 degree 2 poles (-10.1344, 18.2528) (-9.9432, 18.2528) (-9.7584, 18.457) (-9.7001, 18.684) knots 0 0 0 1 2 2 2
  spline S153 degree 2 poles (-9.7001, 18.684) (-9.6709, 18.7942) (-9.6126, 19.0729) (-9.5769, 19.2253) knots 0 0 0 1 2 2 2
  spline S154 degree 2 poles (-9.5769, 19.2253) (-9.4926, 19.5559) (-9.1069, 19.893) (-8.773, 19.893) knots 0 0 0 1 2 2 2
  spline S155 degree 2 poles (-8.773, 19.893) (-8.5785, 19.893) (-8.2349, 19.7407) (-8.1085, 19.5916) knots 0 0 0 1 2 2 2
  spline S156 degree 2 poles (-8.1085, 19.5916) (-7.9756, 19.4327) (-7.8362, 19.0276) (-7.8362, 18.7196) knots 0 0 0 1 2 2 2
  spline S157 degree 2 poles (-7.8395, 21.6661) (-7.8395, 20.9465) (-8.6466, 20.1556) (-9.3921, 20.1556) knots 0 0 0 1 2 2 2
  spline S158 degree 2 poles (-9.3921, 20.1556) (-10.1247, 20.1556) (-10.9934, 20.9238) (-10.9934, 21.5429) knots 0 0 0 1 2 2 2
  spline S159 degree 2 poles (-10.9934, 21.5429) (-10.9934, 21.8217) (-10.8314, 22.2528) (-10.6596, 22.4117) knots 0 0 0 1 2 2 2
  spline S160 degree 2 poles (-10.6596, 22.4117) (-10.4878, 22.5737) (-9.9918, 22.7455) (-9.632, 22.7455) knots 0 0 0 1 2 2 2
  line L114 (-9.632, 22.7455) -> (-9.3565, 22.7455)
  line L115 (-9.3565, 22.7455) -> (-9.3565, 20.6677)
  spline S161 degree 2 poles (-9.3565, 20.6677) (-8.8346, 20.6677) (-8.2803, 21.1929) (-8.2803, 21.6596) knots 0 0 0 1 2 2 2
  spline S162 degree 2 poles (-8.2803, 21.6596) (-8.2803, 21.825) (-8.3549, 22.1459) (-8.4132, 22.2755) knots 0 0 0 1 2 2 2
  spline S163 degree 2 poles (-8.4132, 22.2755) (-8.478, 22.4117) (-8.5915, 22.5997) (-8.6433, 22.6613) knots 0 0 0 1 2 2 2
  line L116 (-8.6433, 22.6613) -> (-8.6433, 22.6904)
  line L117 (-8.6433, 22.6904) -> (-8.0923, 22.6904)
  spline S164 degree 2 poles (-8.0923, 22.6904) (-8.0566, 22.6029) (-7.9529, 22.3371) (-7.9237, 22.2334) knots 0 0 0 1 2 2 2
  spline S165 degree 2 poles (-7.9237, 22.2334) (-7.8816, 22.0875) (-7.8395, 21.8476) (-7.8395, 21.6661) knots 0 0 0 1 2 2 2
  spline S166 degree 2 poles (-9.7422, 22.2528) (-9.9464, 22.2464) (-10.2446, 22.1621) (-10.3451, 22.081) knots 0 0 0 1 2 2 2
  spline S167 degree 2 poles (-10.3451, 22.081) (-10.4586, 21.9935) (-10.5785, 21.718) (-10.5785, 21.5138) knots 0 0 0 1 2 2 2
  spline S168 degree 2 poles (-10.5785, 21.5138) (-10.5785, 21.3128) (-10.4586, 21.0308) (-10.3419, 20.9141) knots 0 0 0 1 2 2 2
  spline S169 degree 2 poles (-10.3419, 20.9141) (-10.222, 20.8006) (-9.9335, 20.684) (-9.7422, 20.6677) knots 0 0 0 1 2 2 2
  line L118 (-9.7422, 20.6677) -> (-9.7422, 22.2528)
  spline S170 degree 2 poles (-10.7017, 27.5429) (-10.4424, 27.5429) (-9.9756, 27.3582) (-9.8135, 27.1929) knots 0 0 0 1 2 2 2
  spline S171 degree 2 poles (-9.8135, 27.1929) (-9.6093, 26.9854) (-9.3986, 26.4246) (-9.3986, 25.9968) knots 0 0 0 1 2 2 2
  line L119 (-9.3986, 25.9968) -> (-9.3986, 25.5462)
  line L120 (-9.3986, 25.5462) -> (-7.9075, 25.5462)
  line L121 (-7.9075, 25.5462) -> (-7.9075, 25.0146)
  line L122 (-7.9075, 25.0146) -> (-11.9075, 25.0146)
  line L123 (-11.9075, 25.0146) -> (-11.9075, 26.0194)
  spline S172 degree 2 poles (-11.9075, 26.0194) (-11.9075, 26.376) (-11.7908, 26.8752) (-11.6579, 27.0665) knots 0 0 0 1 2 2 2
  spline S173 degree 2 poles (-11.6579, 27.0665) (-11.5056, 27.2901) (-11.0356, 27.5429) (-10.7017, 27.5429) knots 0 0 0 1 2 2 2
  spline S174 degree 2 poles (-10.6855, 26.9887) (-10.8929, 26.9887) (-11.1976, 26.846) (-11.2949, 26.7002) knots 0 0 0 1 2 2 2
  spline S175 degree 2 poles (-11.2949, 26.7002) (-11.3792, 26.5737) (-11.4472, 26.2366) (-11.4472, 25.987) knots 0 0 0 1 2 2 2
  line L124 (-11.4472, 25.987) -> (-11.4472, 25.5462)
  line L125 (-11.4472, 25.5462) -> (-9.8524, 25.5462)
  line L126 (-9.8524, 25.5462) -> (-9.8524, 25.9092)
  spline S176 degree 2 poles (-9.8524, 25.9092) (-9.8524, 26.2334) (-9.9562, 26.6321) (-10.0923, 26.7618) knots 0 0 0 1 2 2 2
  spline S177 degree 2 poles (-10.0923, 26.7618) (-10.2122, 26.8817) (-10.4942, 26.9887) (-10.6855, 26.9887) knots 0 0 0 1 2 2 2
  line L127 (-11.9075, 30.9498) -> (-7.9075, 29.5721)
  line L128 (-7.9075, 29.5721) -> (-7.9075, 28.9984)
  line L129 (-7.9075, 28.9984) -> (-11.9075, 27.6207)
  line L130 (-11.9075, 27.6207) -> (-11.9075, 28.1912)
  line L131 (-11.9075, 28.1912) -> (-8.585, 29.2998)
  line L132 (-8.585, 29.2998) -> (-11.9075, 30.4084)
  line L133 (-11.9075, 30.4084) -> (-11.9075, 30.9498)
  line L134 (-7.9075, 35.248) -> (-7.9075, 33.2966)
  line L135 (-7.9075, 33.2966) -> (-8.316, 33.2966)
  line L136 (-8.316, 33.2966) -> (-8.316, 34.0227)
  line L137 (-8.316, 34.0227) -> (-10.9967, 34.0227)
  line L138 (-10.9967, 34.0227) -> (-10.9967, 33.2966)
  line L139 (-10.9967, 33.2966) -> (-11.363, 33.2966)
  spline S178 degree 2 poles (-11.363, 33.2966) (-11.363, 33.7083) (-11.5963, 34.0972) (-11.9205, 34.1232) knots 0 0 0 1 2 2 2
  line L140 (-11.9205, 34.1232) -> (-11.9205, 34.5381)
  line L141 (-11.9205, 34.5381) -> (-8.316, 34.5381)
  line L142 (-8.316, 34.5381) -> (-8.316, 35.248)
  line L143 (-8.316, 35.248) -> (-7.9075, 35.248)
  line L144 (-7.9075, 38.2496) -> (-7.9075, 36.2982)
  line L145 (-7.9075, 36.2982) -> (-8.316, 36.2982)
  line L146 (-8.316, 36.2982) -> (-8.316, 37.0243)
  line L147 (-8.316, 37.0243) -> (-10.9967, 37.0243)
  line L148 (-10.9967, 37.0243) -> (-10.9967, 36.2982)
  line L149 (-10.9967, 36.2982) -> (-11.363, 36.2982)
  spline S179 degree 2 poles (-11.363, 36.2982) (-11.363, 36.7099) (-11.5963, 37.0989) (-11.9205, 37.1248) knots 0 0 0 1 2 2 2
  line L150 (-11.9205, 37.1248) -> (-11.9205, 37.5397)
  line L151 (-11.9205, 37.5397) -> (-8.316, 37.5397)
  line L152 (-8.316, 37.5397) -> (-8.316, 38.2496)
  line L153 (-8.316, 38.2496) -> (-7.9075, 38.2496)
  point P0 (-12, 25)
  constraints: 2 end point, 2 midpoint, 1 vertical
emboss "Emboss2" sketch "Sketch10" operation cut depth 1 direction (-1, 0, 0)
sketch "Sketch11" plane through (0, 0, -12) normal (0, 0, -1) x (-1, 0, 0)
  line L0 (25, -25) -> (25, 25) projected
  line L1 (-25, -25) -> (25, -25) projected
  line L2 (-25, 25) -> (-25, -25) projected
  line L3 (25, 25) -> (-25, 25) projected
  line L4 (-19.75, 19.75) -> (-19.75, -19.75) construction
  line L5 (-19.75, -19.75) -> (19.75, -19.75) construction
  line L6 (19.75, -19.75) -> (19.75, 19.75) construction
  line L7 (19.75, 19.75) -> (-19.75, 19.75) construction
  line L8 (-19.75, 19.75) -> (19.75, -19.75) construction
  line L9 (-19.75, -19.75) -> (19.75, 19.75) construction
  point P0 (0, 0)
  dimension "d74" = 39.5
  dimension "d75" = 39.5
  constraints: 12 end point, 4 coincident, 2 midpoint, 2 parallel, 1 perpendicular, 1 vertical
  measures "d74" distance of L5.end L6.end
  measures "d75" distance of L6.end L4.start
hole "Hole1" at (-19.75, 19.75, -12) at (-19.75, -19.75, -12) at (19.75, -19.75, -12) at (19.75, 19.75, -12) direction (0, 0, 1) diameter 1.6942 end through all thread size "2-56 UNC" class "3B" standard "ANSI Unified Screw Threads"
sketch "Sketch14" plane through (-25, 25, -12) normal (0, 1, 0) x (1, 0, 0)
  line L0 (50, -29) -> (0, -29) projected
  line L1 (50, 0) -> (50, -29) projected
  line L2 (0, 0) -> (50, 0) projected
  line L3 (0, 0) -> (0, -29) projected
  line L4 (50, 0) -> (0, 0) construction
  line L5 (0, 0) -> (0, -29) construction
  line L6 (50, 0) -> (0, -29) construction
  line L7 (50, -29) -> (0, 0) construction
  line L8 (36.547, -16) -> (30.7735, -26)
  line L9 (30.7735, -26) -> (19.2265, -26)
  line L10 (19.2265, -26) -> (13.453, -16)
  line L11 (13.453, -16) -> (19.2265, -6)
  line L12 (19.2265, -6) -> (30.7735, -6)
  line L13 (30.7735, -6) -> (36.547, -16)
  point P0 (25, -12)
  point P1 (25, -16)
  dimension "d101" = 20
  constraints: 16 end point, 1 horizontal, 13 other
  measures "d101" distance between parallel lines of L9 L12
sketch "Sketch15" plane through (-25, 25, -12) normal (0, 1, 0) x (1, 0, 0)
  line L0 (0, 0) -> (50, 0) projected
  line L1 (50, 0) -> (50, -29) projected
  line L2 (50, -29) -> (0, -29) projected
  line L3 (0, 0) -> (0, -29) projected
  line L4 (0, 0) -> (50, -29) construction
  line L5 (50, 0) -> (0, -29) construction
  line L6 (13.1, -26.4) -> (36.9, -26.4) construction
  line L7 (36.9, -26.4) -> (36.9, -2.6) construction
  line L8 (36.9, -2.6) -> (13.1, -2.6) construction
  line L9 (13.1, -2.6) -> (13.1, -26.4) construction
  line L10 (13.1, -26.4) -> (36.9, -2.6) construction
  line L11 (36.9, -26.4) -> (13.1, -2.6) construction
  point P0 (25, -12)
  point P1 (25, -14.5)
  dimension "d93" = 23.8
  constraints: 16 end point, 4 coincident, 3 midpoint, 2 parallel, 2 perpendicular, 1 horizontal
  measures "d93" distance of L8.end L6.start
hole "Hole3" at (-11.9, 25, -9.4) at (11.9, 25, -9.4) at (11.9, 25, 14.4) at (-11.9, 25, 14.4) direction (0, -1, 0) diameter 1.6942 depth 4 thread size "2-56 UNC" class "2B" standard "ANSI Unified Screw Threads"
extrude "Extrusion13" cut sketch "Sketch14" against normal through all contours L8 L9 L10 L11 L12 L13
equation "\"d46\" = screwSpacing"
equation "\"d47\" = screwSpacing"
equation "\"d48\" = holeDiameter"
equation "\"d49\" = interiorWidth"
equation "\"d50\" = interiorWidth"
equation "\"d51\" = sideWallThickness"
equation "\"d52\" = sideWallThickness"
equation "\"d101\" = hexCoolingHole"
equation "\"screwSpacing\" = 34"
equation "\"interiorWidth\" = 42"
equation "\"bottomWallThickness\" = 2"
equation "\"holeDiameter\" = 1.8"
equation "\"sideWallThickness\" = 4"
equation "\"hexCoolingHole\" = 20"
body "Solid4"
body "Solid5"
